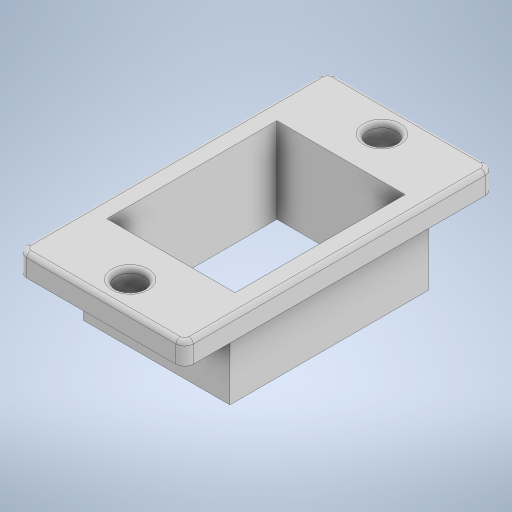
# Autodesk Inventor part: Delock_86213_Grob
Saved by Autodesk Inventor 2024.2 (Build 282272000, 272)
## iProperties
Created: 2024-04-15
Part Number: Delock_86213_Grob
Material: Generisch
Document SubType Name: Modeling
Designer: Holger
Density: 1 g/cm^3
Appearance: Vorgabe
Author: Holger
Autodesk Inventor part; units mm, degrees
ref_plane "YZ Plane" through (0, 0, 0) normal (1, 0, 0) x (0, 1, 0)
ref_plane "XZ Plane" through (0, 0, 0) normal (0, 1, 0) x (-1, 0, 0)
ref_plane "XY Plane" through (0, 0, 0) normal (0, 0, 1) x (1, 0, 0)
sketch "Skizze1" plane through (0, 0, 0) normal (0, 0, 1) x (1, 0, 0)
  line L0 (-8.4, 11.4) -> (8.4, 11.4)
  line L1 (8.4, 11.4) -> (8.4, -11.4)
  line L2 (8.4, -11.4) -> (-8.4, -11.4)
  line L3 (-8.4, -11.4) -> (-8.4, 11.4)
  line L4 (-13.6739, 0) -> (13.6739, 0) projected
  line L5 (0, -25.1399) -> (0, 25.1399) projected
  line L6 (-7.35, 9.75) -> (7.35, 9.75)
  line L7 (7.35, 9.75) -> (7.35, -9.75)
  line L8 (7.35, -9.75) -> (-7.35, -9.75)
  line L9 (-7.35, -9.75) -> (-7.35, 9.75)
  line L10 (-8.56, 17.75) -> (8.56, 17.75)
  line L11 (9.56, 16.75) -> (9.56, -16.75)
  line L12 (8.56, -17.75) -> (-8.56, -17.75)
  line L13 (-9.56, -16.75) -> (-9.56, 16.75)
  circle A0 centre (0, 14.45) radius 1.6
  line L14 (-9.56, -17.75) -> (9.56, -17.75)
  circle A1 centre (0, -14.45) radius 1.6
  arc A2 (-8.56, 17.75) -> (-9.56, 16.75) centre (-8.56, 16.75) ccw
  arc A3 (9.56, 16.75) -> (8.56, 17.75) centre (8.56, 16.75) ccw
  arc A4 (8.56, -17.75) -> (9.56, -16.75) centre (8.56, -16.75) ccw
  arc A5 (-9.56, -16.75) -> (-8.56, -17.75) centre (-8.56, -16.75) ccw
  point P0 (0, 0)
  point P1 (-9.56, 17.75)
  point P2 (9.56, 17.75)
  dimension "d0" = 16.8
  dimension "d1" = 22.8
  dimension "d2" = 19.5
  dimension "d3" = 14.7
  dimension "d4" = 35.5
  dimension "d5" = 19.12
  dimension "d6" = 3.2
  dimension "d7" = 28.9
  dimension "d8" = 1
  constraints: 26 end point, 9 point on line, 8 point on circle, 8 tangent, 6 centre point, 6 parallel, 3 equal radius, 3 horizontal, 3 perpendicular, 1 symmetric about line, 7 other
  measures "d0" distance of L0.start L0.end
  measures "d1" distance of L2.end L0.start
  measures "d2" distance of L8.end L6.start
  measures "d3" distance of L6.start L6.end
  measures "d4" distance of L14.start point (-9.56, 17.75)
  measures "d5" distance of point (-9.56, 17.75) point (9.56, 17.75)
  measures "d6" diameter of A0
  measures "d7" distance of A1.centre A0.centre
  measures "d8" radius of A2
extrude "Extrusion1" add sketch "Skizze1" against normal blind 7.3 contours L0 L5 L6 L9 L4 L3 | L0 L1 L4 L7 L6 L5 | L4 L9 L8 L5 L2 L3 | L1 L2 L5 L8 L7 L4
extrude "Extrusion2" add sketch "Skizze1" along normal blind 2.5 contours L3 L4 L13 A2 L10 L5 A0 L0 | L0 L5 L6 L9 L4 L3 | L5 A0 L10 A3 L11 L4 L1 L0 | L0 L1 L4 L7 L6 L5 | L4 L9 L8 L5 L2 L3 | L3 L2 L5 A1 L12 A5 L13 L4 | L4 L11 A4 L12 L5 A1 L2 L1 | L1 L2 L5 L8 L7 L4
fillet "Rundung1" radius 0.5 10 edges at (-9.2671, 17.4571, 2.5) (-9.56, 0, 2.5) (-9.2671, -17.4571, 2.5) (0, -17.75, 2.5) (9.2671, -17.4571, 2.5) (9.56, 0, 2.5) (9.2671, 17.4571, 2.5) (0, 17.75, 2.5) (-1.6, 14.45, 2.5) (-1.6, -14.45, 2.5)
